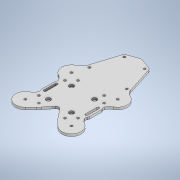
# Autodesk Inventor part: 399 prig z plate
Saved by Autodesk Inventor 2020 (Build 240168000, 168)
## iProperties
Created: 2022-05-23
Part Number: 399 prig z plate
Material: Generic
Document SubType Name: Modeling
Designer: Steven
Density: 1 g/cm^3
Appearance: Default
Author: Steven
Autodesk Inventor part; units mm, degrees
ref_plane "YZ Plane" through (0, 0, 0) normal (1, 0, 0) x (0, 1, 0)
ref_plane "XZ Plane" through (0, 0, 0) normal (0, 1, 0) x (-1, 0, 0)
ref_plane "XY Plane" through (0, 0, 0) normal (0, 0, 1) x (1, 0, 0)
sketch "Sketch1" plane through (0, 0, 0) normal (0, 1, 0) x (-1, 0, 0)
  arc A0 (-30.0072, 97.3212) -> (-35.8309, 103.5589) centre (-41.895, 92.0599) ccw
  arc A1 (-30.286, 94.3964) -> (-30.0072, 97.3212) centre (-32.7505, 96.107) ccw
  arc A2 (-30.286, 94.3964) -> (-31, 92.1156) centre (-27, 92.1156) ccw
  line L0 (-31, 92.1156) -> (-31, 77.1156)
  arc A3 (-31, 77.1156) -> (-30.286, 74.8348) centre (-27, 77.1156) ccw
  arc A4 (-30.0072, 71.9101) -> (-30.286, 74.8348) centre (-32.7505, 73.1242) ccw
  arc A5 (-35.8309, 65.6723) -> (-30.0072, 71.9101) centre (-41.895, 77.1713) ccw
  arc A6 (-35.8309, 65.6723) -> (-34.9925, 43.1559) centre (-30, 54.6156) ccw
  arc A7 (-27.7949, 35.1735) -> (-34.9925, 43.1559) centre (-40.1848, 31.2379) ccw
  line L1 (-27.7949, 35.1735) -> (-17.0958, 1.4913)
  arc A8 (-17.0958, 1.4913) -> (-14.6505, -1.0569) centre (-13.2835, 2.7022) ccw
  line L2 (-14.6505, -1.0569) -> (-2.0505, -5.6388)
  arc A9 (-2.0505, -5.6388) -> (2.0505, -5.6388) centre (0, 0) ccw
  line L3 (2.0505, -5.6388) -> (14.6505, -1.0569)
  arc A10 (14.6505, -1.0569) -> (17.0958, 1.4913) centre (13.2835, 2.7022) ccw
  line L4 (17.0958, 1.4913) -> (27.7949, 35.1735)
  arc A11 (34.9925, 43.1559) -> (27.7949, 35.1735) centre (40.1848, 31.2379) ccw
  arc A12 (34.9925, 43.1559) -> (35.8309, 65.6723) centre (30, 54.6156) ccw
  arc A13 (30.0072, 71.9101) -> (35.8309, 65.6723) centre (41.895, 77.1713) ccw
  arc A14 (30.286, 74.8348) -> (30.0072, 71.9101) centre (32.7505, 73.1242) ccw
  arc A15 (30.286, 74.8348) -> (31, 77.1156) centre (27, 77.1156) ccw
  line L5 (31, 77.1156) -> (31, 92.1156)
  arc A16 (31, 92.1156) -> (30.286, 94.3964) centre (27, 92.1156) ccw
  arc A17 (30.0072, 97.3212) -> (30.286, 94.3964) centre (32.7505, 96.107) ccw
  arc A18 (35.8309, 103.5589) -> (30.0072, 97.3212) centre (41.895, 92.0599) ccw
  arc A19 (35.8309, 103.5589) -> (21.1612, 123.4545) centre (30, 114.6156) ccw
  line L6 (21.1612, 123.4545) -> (13.9152, 116.2085)
  arc A20 (13.9152, 116.2085) -> (11.0366, 112.9476) centre (38.6639, 91.4597) ccw
  line L7 (11.0366, 112.9476) -> (3.1574, 102.8173)
  arc A21 (-3.1574, 102.8173) -> (3.1574, 102.8173) centre (0, 105.273) ccw
  line L8 (-3.1574, 102.8173) -> (-11.0366, 112.9476)
  arc A22 (-11.0366, 112.9476) -> (-13.9152, 116.2085) centre (-38.6639, 91.4597) ccw
  line L9 (-13.9152, 116.2085) -> (-21.1612, 123.4545)
  arc A23 (-21.1612, 123.4545) -> (-35.8309, 103.5589) centre (-30, 114.6156) ccw
  arc A24 (25.5, 77.1156) -> (28.5, 77.1156) centre (27, 77.1156) ccw
  line L10 (25.5, 92.1156) -> (25.5, 77.1156)
  arc A25 (28.5, 92.1156) -> (25.5, 92.1156) centre (27, 92.1156) ccw
  line L11 (28.5, 77.1156) -> (28.5, 92.1156)
  arc A26 (-28.5, 77.1156) -> (-25.5, 77.1156) centre (-27, 77.1156) ccw
  line L12 (-28.5, 92.1156) -> (-28.5, 77.1156)
  arc A27 (-25.5, 92.1156) -> (-28.5, 92.1156) centre (-27, 92.1156) ccw
  line L13 (-25.5, 77.1156) -> (-25.5, 92.1156)
  circle A28 centre (-30, 54.6156) radius 1.5
  circle A29 centre (-13.2835, 2.7022) radius 1.5
  circle A30 centre (-25.4558, 101.5862) radius 1.5
  circle A31 centre (-25.4558, 67.6451) radius 1.5
  circle A32 centre (-15, 99.6156) radius 3
  circle A33 centre (25.4558, 67.6451) radius 1.5
  circle A34 centre (25.4558, 101.5862) radius 1.5
  circle A35 centre (15, 69.6156) radius 3
  circle A36 centre (30, 54.6156) radius 1.5
  circle A37 centre (30, 114.6156) radius 1.5
  circle A38 centre (24.2029, 37.0782) radius 1.5
  circle A39 centre (13.2835, 2.7022) radius 1.5
  circle A40 centre (16.9706, 110.0715) radius 1.5
  circle A41 centre (16.9706, 59.1598) radius 1.5
  circle A42 centre (15, 99.6156) radius 3
  circle A43 centre (-15, 69.6156) radius 3
  circle A44 centre (-16.9706, 59.1598) radius 1.5
  circle A45 centre (-16.9706, 110.0715) radius 1.5
  circle A46 centre (-24.2029, 37.0782) radius 1.5
  circle A47 centre (-30, 114.6156) radius 1.5
  point P0 (-30.286, 94.3964)
  point P1 (-35.8309, 65.6723)
  point P2 (-34.9925, 43.1559)
  point P3 (-27.7949, 35.1735)
  point P4 (-17.0958, 1.4913)
  point P5 (-14.6505, -1.0569)
  point P6 (2.0505, -5.6388)
  point P7 (14.6505, -1.0569)
  point P8 (27.7949, 35.1735)
  point P9 (35.8309, 65.6723)
  point P10 (30.0072, 71.9101)
  point P11 (30.286, 74.8348)
  point P12 (30.286, 94.3964)
  point P13 (30.0072, 97.3212)
  point P14 (13.9152, 116.2085)
  point P15 (11.0366, 112.9476)
  point P16 (-3.1574, 102.8173)
  point P17 (-13.9152, 116.2085)
  point P18 (-21.1612, 123.4545)
  point P19 (-35.8309, 103.5589)
  point P20 (-30.0072, 97.3212)
  point P21 (25.5, 77.1156)
  point P22 (28.5, 77.1156)
  constraints: 56 point on circle, 48 centre point, 28 end point
extrude "Extrusion1" add sketch "Sketch1" along normal blind 3
body "Solid1"
